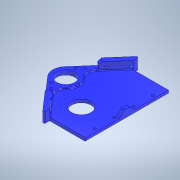
# Autodesk Inventor part: Motor Mount top
Saved by Autodesk Inventor 2022 (Build 260153000, 153)
## iProperties
Created: 2022-08-10
Part Number: Motor Mount top
Material: Generic
Document SubType Name: Modeling
Designer: Nick
Density: 1 g/cm^3
Appearance: Blue - Wall Paint - Glossy
Mass: 61.7644 g
Surface Area: 281.958 cm^2
Volume: 61.7644 cm^3
Author: Nick
Autodesk Inventor part; units mm, degrees
ref_plane "YZ Plane" through (0, 0, 0) normal (1, 0, 0) x (0, 1, 0)
ref_plane "XZ Plane" through (0, 0, 0) normal (0, 1, 0) x (-1, 0, 0)
ref_plane "XY Plane" through (0, 0, 0) normal (0, 0, 1) x (1, 0, 0)
sketch "Sketch14" plane through (0, 0, 0) normal (0, 0, 1) x (1, 0, 0)
  line L0 (0, 0) -> (55, 0)
  line L1 (55, 0) -> (55, 45)
  line L2 (55, 45) -> (0, 45)
  line L3 (0, 45) -> (0, 0)
  circle A0 centre (27.5, 22.5) radius 12.25
  point P0 (55, 22.5)
  point P1 (27.5, 45)
  dimension "d94" = 24.5
  dimension "d95" = 55
  dimension "d96" = 45
  constraints: 8 end point, 2 midpoint, 2 parallel, 1 centre point, 1 horizontal, 1 horizontal alignment, 1 perpendicular, 1 vertical alignment
  measures "d94" diameter of A0
  measures "d95" distance of L0.start L0.end
  measures "d96" distance of L2.end L0.start
extrude "Extrusion13" add sketch "Sketch14" along normal blind 11.26
sketch "Sketch15" plane through (0, 0, 0) normal (0, -1, 0) x (1, 0, 0)
  line L0 (0, 0) -> (55, 0) projected
  line L1 (55, 0) -> (55, 11.26) projected
  line L2 (0, 11.26) -> (55, 11.26) projected
  line L3 (0, 0) -> (0, 11.26) projected
  line L4 (55, 0) -> (55, 11.26) projected
  line L5 (55, 11.26) -> (0, 11.26)
  line L6 (0, 11.26) -> (0, 76.185)
  line L7 (0, 76.185) -> (55, 76.185)
  line L8 (55, 76.185) -> (55, 11.26)
  line L9 (0, 0) -> (0, 11.26) projected
  point P0 (0, 11.26)
  dimension "d99" = 64.925
  constraints: 8 end point, 2 parallel, 1 collinear, 1 horizontal, 1 perpendicular
  measures "d99" distance of L7.end L1.end
extrude "Extrusion14" add sketch "Sketch15" against normal blind 5 contours L6 L7 L8 L2
mirror "Mirror4" about plane through (0, 0, 76.185) normal (0, 0, 1)
sketch "Sketch26" plane through (0, 0, 0) normal (0, -1, 0) x (1, 0, 0)
  line L0 (0, 0) -> (55, 0) projected
  line L1 (0, 0) -> (-55.0618, 63.0266)
  line L2 (0, 152.37) -> (-55.0618, 89.3434)
  arc A0 (-55.0618, 89.3434) -> (-55.0618, 63.0266) centre (-40, 76.185) ccw
  line L3 (0, 0) -> (0, 152.37) projected
  line L4 (0, 0) -> (0, 152.37)
  circle A1 centre (-40, 76.185) radius 14
  point P0 (0, 44.2511)
  point P1 (0, 44.2511)
  dimension "d137" = 20
  dimension "d138" = 40
  dimension "d146" = 28
  constraints: 6 end point, 2 centre point, 2 point on circle, 2 tangent, 1 coincident, 1 equal length, 1 vertical
  measures "d137" radius of A0
  measures "d138" distance from line of L3 A0.centre
  measures "d146" diameter of A1
extrude "Extrusion25" add sketch "Sketch26" against normal blind 5
sketch "Sketch27" plane through (0, 5, 0) normal (0, 1, 0) x (1, 0, 0)
  arc A0 (-55.0618, -63.0266) -> (-55.0618, -89.3434) centre (-40, -76.185) ccw projected
  circle A1 centre (-40, -76.185) radius 14
  circle A2 centre (-40, -76.185) radius 20
  line L0 (0, 0) -> (-55.0618, -63.0266) projected
  line L1 (-55.0618, -89.3434) -> (0, -152.37) projected
  line L2 (55, -141.11) -> (0, -141.11) projected
  line L3 (-26.5102, -110.765) -> (0, -141.11)
  line L4 (0, -11.26) -> (-26.5102, -41.605)
  arc A3 (-26.5102, -41.605) -> (-25.8365, -62.0643) centre (-15.2138, -51.4737) ccw
  arc A4 (-25.8365, -90.3057) -> (-26.5102, -110.765) centre (-15.2138, -100.8963) ccw
  line L5 (-55.0618, -63.0266) -> (0, 0) projected
  line L6 (0, 0) -> (0, -11.26)
  line L7 (0, -141.11) -> (55, -141.11) projected
  line L8 (0, -152.37) -> (0, -141.11) projected
  line L9 (0, -141.11) -> (0, -152.37)
  point P0 (-32.2708, -36.9389)
  point P1 (-29.1283, -59.3979)
  point P2 (-29.1283, -92.9721)
  point P3 (-32.2708, -115.4311)
  point P4 (3, -141.11)
  point P5 (12, -141.11)
  point P6 (-55.0618, -63.0266)
  point P7 (52, -141.11)
  point P8 (51, -141.11)
  dimension "d141" = 28
  dimension "d145" = 15
  constraints: 9 point on circle, 8 end point, 4 centre point, 4 tangent, 2 coincident, 2 parallel, 2 point on line, 1 collinear, 1 equal radius, 1 vertical
  measures "d141" diameter of A1
  measures "d145" radius of A3
extrude "Extrusion26" add sketch "Sketch27" along normal blind 2
sketch "Sketch29" plane through (0, 5, 0) normal (0, 1, 0) x (1, 0, 0)
  line L0 (50, -11.26) -> (3, -11.26) projected
  circle A0 centre (10, -102.11) radius 15
  line L1 (55, -141.11) -> (0, -141.11) projected
  line L2 (55, -11.26) -> (55, -141.11) projected
  point P0 (0, 0)
  dimension "d151" = 30
  dimension "d202" = 39
  dimension "d203" = 45
  constraints: 1 centre point
  measures "d151" diameter of A0
  measures "d202" distance from line of A0.centre L1
  measures "d203" distance from line of L2 A0.centre
extrude "Extrusion28" cut sketch "Sketch29" against normal blind 10
sketch "Sketch37" plane through (0, 5, 0) normal (0, 1, 0) x (1, 0, 0)
  circle A0 centre (10, -102.11) radius 15 projected
  line L0 (-26.5102, -110.765) -> (0, -141.11) projected
  line L1 (0, -141.11) -> (55, -141.11) projected
  line L2 (55, -11.26) -> (55, -141.11) projected
  line L3 (0, -11.26) -> (55, -11.26) projected
  line L4 (0, -11.26) -> (-26.5102, -41.605) projected
  arc A1 (-26.5102, -41.605) -> (-25.8365, -62.0643) centre (-15.2138, -51.4737) ccw projected
  arc A2 (-25.8365, -90.3057) -> (-25.8365, -62.0643) centre (-40, -76.185) ccw projected
  arc A3 (-25.8365, -90.3057) -> (-26.5102, -110.765) centre (-15.2138, -100.8963) ccw projected
  line L5 (0, -141.11) -> (-26.5102, -110.765) projected
  line L6 (0, -152.37) -> (0, -141.11) projected
  line L7 (0, -141.11) -> (0, -152.37)
  line L8 (55, 0) -> (0, 0) projected
  line L9 (0, -11.26) -> (0, 0)
  line L10 (0, -152.37) -> (55, -152.37) projected
  line L11 (55, 0) -> (55, -11.26) projected
  line L12 (0, -152.37) -> (55, -152.37)
  line L13 (55, -152.37) -> (55, 0)
  line L14 (55, 0) -> (0, 0)
  line L15 (0, 0) -> (0, -152.37)
  point P0 (0, -90.9297)
  point P1 (0, -113.2903)
  point P2 (0, -141.11)
  constraints: 12 end point, 3 equal length, 1 horizontal, 1 perpendicular, 1 vertical
extrude "Extrusion35" cut sketch "Sketch37" along normal through all contours A0 L15 | A0 L15 L3 L2 L1 | L9 L8 L11 L3 | L1 L13 L10 L6 picked at (7.1891, -98.9267)
sketch "Sketch40" plane through (0, 5, 0) normal (0, 1, 0) x (1, 0, 0)
  circle A0 centre (10, -102.11) radius 15 projected
  line L0 (0, -11.26) -> (-26.5102, -41.605) projected
  arc A1 (-26.5102, -41.605) -> (-25.8365, -62.0643) centre (-15.2138, -51.4737) ccw projected
  arc A2 (-25.8365, -90.3057) -> (-25.8365, -62.0643) centre (-40, -76.185) ccw projected
  arc A3 (-25.8365, -90.3057) -> (-26.5102, -110.765) centre (-15.2138, -100.8963) ccw projected
  line L1 (-26.5102, -110.765) -> (0, -141.11) projected
  line L2 (0, -141.11) -> (0, -152.37) projected
  line L3 (55, -152.37) -> (0, -152.37) projected
  line L4 (55, 0) -> (55, -152.37) projected
  line L5 (0, 0) -> (55, 0) projected
  line L6 (0, 0) -> (0, -11.26) projected
  line L7 (55, 0) -> (0, 0)
  line L8 (0, 0) -> (0, -12)
  line L9 (0, -12) -> (55, -12)
  line L10 (55, -12) -> (55, 0)
  line L11 (55, -152.37) -> (55, 0) projected
  line L12 (55, -152.37) -> (0, -152.37)
  line L13 (0, -152.37) -> (0, -140.37)
  line L14 (0, -140.37) -> (55, -140.37)
  line L15 (55, -140.37) -> (55, -152.37)
  point P0 (0, -141.11)
  dimension "d198" = 12
  dimension "d199" = 12
  constraints: 16 end point, 4 parallel, 2 horizontal, 2 perpendicular, 2 point on line
  measures "d198" distance of L8.end L7.end
  measures "d199" distance of L12.end L13.end
extrude "Extrusion38" cut sketch "Sketch40" against normal through all contours L6 L5 L4 L9 L8 | L4 L3 L2 L13 L14
sketch "Sketch41" plane through (0, 7, 0) normal (0, 1, 0) x (1, 0, 0)
  line L0 (-26.5102, -41.605) -> (0, -11.26) projected
  line L1 (0, -11.26) -> (-5.579, -6.386)
  line L2 (0, 0) -> (-55.0618, -63.0266) projected
  line L3 (-25.3432, -40.2691) -> (-30.9222, -35.3952)
  line L4 (0, 0) -> (0, -11.26) projected
  line L5 (0, -11.26) -> (0, 0)
  arc A0 (-25.8365, -90.3057) -> (-25.8365, -62.0643) centre (-40, -76.185) ccw projected
  arc A1 (-26.5102, -41.605) -> (-25.8365, -62.0643) centre (-15.2138, -51.4737) ccw projected
  line L6 (-26.5102, -41.605) -> (0, -11.26) projected
  line L7 (0, 0) -> (0, -11.26) projected
  line L8 (0, 0) -> (-55.0618, -63.0266) projected
  arc A2 (-55.0618, -63.0266) -> (-55.0618, -89.3434) centre (-40, -76.185) ccw projected
  line L9 (-55.0618, -89.3434) -> (0, -152.37) projected
  line L10 (0, -141.11) -> (0, -152.37) projected
  line L11 (0, -141.11) -> (-26.5102, -110.765) projected
  arc A3 (-25.8365, -90.3057) -> (-26.5102, -110.765) centre (-15.2138, -100.8963) ccw projected
  circle A4 centre (-40, -76.185) radius 14 projected
  line L12 (0, -141.11) -> (-5.579, -145.984)
  line L13 (0, -152.37) -> (-55.0618, -89.3434) projected
  line L14 (0, -141.11) -> (-26.5102, -110.765) projected
  line L15 (-25.3432, -112.1009) -> (-30.9222, -116.9748)
  line L16 (0, -140.37) -> (0, -152.37) projected
  line L17 (0, -152.37) -> (0, -141.11)
  point P0 (-25.3432, -40.2691)
  point P1 (-25.3432, -112.1009)
  dimension "d204" = 47
  dimension "d207" = 47
  constraints: 12 end point, 5 point on line, 3 perpendicular, 1 collinear, 1 parallel, 1 vertical
  measures "d204" distance of L3.end L2.start
  measures "d207" distance from line of L9.end L15
extrude "Extrusion39" add sketch "Sketch41" along normal blind 10 contours L3 L2 L1 L0 | L1 L2 L4 | L11 L12 L9 L15 | L10 L9 L12
sketch "Sketch42" plane through (-40, 0, 76.185) normal (0, -1, 0) x (1, 0, 0)
  line L0 (95, 64.185) -> (40, 64.185) projected
  line L1 (40, 64.185) -> (40, 76.185) projected
  line L2 (40, 76.185) -> (-15.0618, 13.1584) projected
  arc A0 (-15.0618, 13.1584) -> (-15.0618, -13.1584) centre (0, 0) ccw projected
  line L3 (-15.0618, -13.1584) -> (40, -76.185) projected
  line L4 (40, -76.185) -> (40, -64.185) projected
  line L5 (40, -64.185) -> (95, -64.185) projected
  line L6 (95, 64.185) -> (95, -64.185) projected
  circle A1 centre (0, 0) radius 14 projected
  circle A2 centre (50, 25.925) radius 15 projected
  line L7 (42.7951, -64.185) -> (6.8232, -23.0096) construction
  line L8 (85, 54.185) -> (85, -54.185) construction
  line L9 (6.8232, 23.0096) -> (34.0588, 54.185) construction
  arc A3 (6.8232, -23.0096) -> (6.8232, 23.0096) centre (0, 0) ccw construction
  line L10 (6.8232, -23.0096) -> (-0.7077, -29.5888) construction
  line L11 (21.9553, -40.3307) -> (14.4245, -46.9099) construction
  line L12 (37.0875, -57.6517) -> (29.5566, -64.2309) construction
  circle A4 centre (0, 0) radius 19 construction
  line L13 (-3.6237, -18.6512) -> (3.0578, -26.2992) construction
  line L14 (8.495, 24.9233) -> (0.9641, 31.5025) construction
  line L15 (40, 76.185) -> (-15.0618, 13.1584) construction
  line L16 (4.7296, 28.2129) -> (-3.6237, 18.6512) construction
  line L17 (0, 0) -> (14, 0) construction
  line L18 (85, 0) -> (95, 0) construction
  line L19 (95, -64.185) -> (95, 64.185) projected
  point P0 (18.1899, -43.6203)
  point P1 (33.322, -60.9413)
  point P2 (19, 0)
  point P3 (33.322, -60.9413)
  point P4 (18.1899, -43.6203)
  point P5 (3.0578, 26.2992)
  point P6 (18.1899, 43.6203)
  point P7 (33.322, 60.9413)
  point P8 (90, 45)
  point P9 (90, 15)
  point P10 (90, -15)
  point P11 (90, -45)
  point P12 (90, 0)
  dimension "d208" = 10
  dimension "d210" = 24
  dimension "d211" = 10
  dimension "d213" = 10
  dimension "d214" = 23
  dimension "d215" = 23
  dimension "d216" = 5
  dimension "d217" = 5
  dimension "d220" = 30
  dimension "d222" = 30
  dimension "d223" = 19.185
  dimension "d224" = 19.185
  dimension "d225" = 30
  constraints: 22 end point, 8 point on line, 7 midpoint, 6 perpendicular, 5 coincident, 5 point on circle, 4 vertical alignment, 3 symmetric about line, 2 centre point, 2 horizontal alignment, 1 horizontal, 1 other
  measures "d208" distance between parallel lines of L3 L7
  measures "d210" radius of A3
  measures "d211" distance between parallel lines of L2 L9
  measures "d213" distance between parallel lines of L6 L8
  measures "d214" distance between parallel lines of L11 L10
  measures "d215" distance between parallel lines of L12 L11
  measures "d216" radial gap between concentric circles of A3 A4
  measures "d220" distance of point (90, 15) point (90, 45)
  measures "d222" distance of point (90, -45) point (90, -15)
  measures "d223" distance from line of point (90, 45) L0
  measures "d224" distance from line of L5 point (90, -45)
  measures "d225" distance of point (90, -15) point (90, 15)
hole "Hole5" at (-36.9422, 0, 49.8858) at (-21.8101, 0, 32.5647) at (-6.678, 0, 15.2437) at (-21, 0, 76.185) at (-43.6237, 0, 57.5338) at (-43.6237, 0, 94.8362) at (-36.9422, 0, 102.4842) at (-21.8101, 0, 119.8053) at (-6.678, 0, 137.1263) at (50, 0, 121.185) at (50, 0, 91.185) at (50, 0, 61.185) at (50, 0, 31.185) direction (0, 1, 0) diameter 4 depth 7
fillet "Fillet3" radius 2 6 edges at (0, 2.5, 0) (0, 6, 0) (0, 12, 0) (0, 2.5, 152.37) (0, 6, 152.37) (0, 12, 152.37)
fillet "Fillet4" radius 1 12 edges at (-30.2057, 5, 100.4026) (-21.8743, 5, 84.6383) (-13.2551, 5, 125.9375) (-30.2057, 5, 51.9674) (-13.2551, 5, 26.4325) (-21.8743, 5, 67.7317) (-30.2057, 7, 51.9674) (-25.9267, 7, 40.937) (-21.8743, 7, 67.7317) (-30.2057, 7, 100.4026) (-25.9267, 7, 111.433) (-21.8743, 7, 84.6383)
sketch "Sketch43" plane through (-55.0618, 0, 89.3434) normal (-0.7530888, 0, 0.6579189) x (0.6579189, 0, 0.7530888)
  ellipse E0 centre (45.4474, 9) end of major axis (45.4474, 7.3) minor radius 1.7 projected
  ellipse E1 centre (72.4474, 9) end of major axis (72.4474, 7.3) minor radius 1.7 projected
  point P0 (-31.0573, 0)
  constraints: 2 other
hole "Hole6" at (-25.1611, 9, 123.5693) at (-7.3973, 9, 143.9027) direction (0.7530888, 0, -0.6579189) diameter 4 depth 8 tip angle 118
sketch "Sketch44" plane through (-55.0618, 0, 63.0266) normal (-0.7530888, 0, -0.6579189) x (-0.6579189, 0, 0.7530888)
  ellipse E0 centre (-45.4248, 9) end of major axis (-45.4248, 7.3) minor radius 1.7 projected
  ellipse E1 centre (-72.4248, 9) end of major axis (-72.4248, 7.3) minor radius 1.7 projected
  point P0 (-83.6908, 0)
hole "Hole7" at (-7.4122, 9, 8.4843) at (-25.176, 9, 28.8177) direction (0.7530888, 0, 0.6579189) diameter 4 depth 8 tip angle 118
chamfer "Chamfer3" distance 1 angle 45 10 edges at (-29.284, 0, 118.85) (-60, 0, 76.185) (-29.284, 0, 33.52) (-1.2973, 0, 3.4567) (0, 0, 8.2946) (0, 0, 11.63) (-1.2973, 0, 148.9133) (0, 0, 144.0754) (0, 0, 140.74) (55, 0, 76.185)
chamfer "Chamfer4" distance 4 angle 45 2 edges at (-28.1327, 17, 114.5378) (-28.1327, 17, 37.8322)
sketch "Sketch45" plane through (55, 5, 140.37) normal (1, 0, 0) x (0, 0, -1)
  line L0 (52.785, 0) -> (60.185, 7.4)
  line L1 (60.185, 7.4) -> (68.185, 7.4)
  line L2 (68.185, 7.4) -> (75.585, 0)
  line L3 (128.37, 0) -> (0, 0) projected
  point P0 (140.37, -5)
  point P1 (64.185, 0)
  point P2 (64.185, 7.4)
  dimension "d255" = 7.4
  dimension "d256" = 8
  dimension "d257" = 135
  constraints: 6 end point, 2 midpoint, 2 point on line, 1 horizontal, 1 perpendicular, 1 vertical alignment
  measures "d255" distance between parallel lines of L3 L1
  measures "d256" distance of L0.end L1.end
  measures "d257" angle of L1 L2
extrude "Extrusion40" add sketch "Sketch45" against normal blind 5
body "Solid3"
